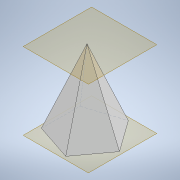
# Autodesk Inventor part: smallPart
Saved by Autodesk Inventor 2021 (Build 250183000, 183)
## iProperties
Created: 2020-11-29
Part Number: smallPart
Material: Generic
Document SubType Name: Modeling
Designer: awitc
Density: 1 g/cm^3
Appearance: Default
Author: awitc
Autodesk Inventor part; units mm, degrees
ref_plane "YZ Plane" through (0, 0, 0) normal (1, 0, 0) x (0, 1, 0)
ref_plane "XY Plane" through (0, 0, 0) normal (0, 0, 1) x (1, 0, 0)
sketch "Sketch1" plane through (0, 0, 0) normal (0, 1, 0) x (-1, 0, 0)
  line L0 (20.5552, -15.1238) -> (-8.0316, -24.2227)
  line L1 (-8.0316, -24.2227) -> (-25.5191, 0.1533)
  line L2 (-25.5191, 0.1533) -> (-7.74, 24.3175)
  line L3 (-7.74, 24.3175) -> (20.7355, 14.8757)
  line L4 (20.7355, 14.8757) -> (20.5552, -15.1238)
  point P0 (0, 0)
  constraints: 10 end point, 11 other
ref_plane "Work Plane1" through (0, 60, 0) normal (0, 1, 0) x (-1, 0, 0)
sketch "Sketch2" plane through (0, 60, 0) normal (0, 1, 0) x (-1, 0, 0)
  point P0 (0, 0)
  point P1 (0, 0)
  constraints: 1 coincident
loft "Loft1" add profiles "Sketch1" section 2 point at (0, 60, 0)
body "Solid1"
